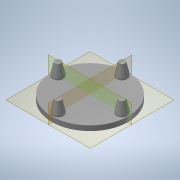
# Autodesk Inventor part: Kogel houder2
Saved by Autodesk Inventor 2021 (Build 250183000, 183)
## iProperties
Manager: PJ / DCS
Company: Emmaüs Bovenbouw Aalter
Created: 2021-02-11
Part Number: Kogel houder2
Material: S235
Catalog Web Link: http://emmausbovenbouw.op-weg.be/
Vendor: Emmaüsinstituut Bovenbouw Aalter
Document SubType Name: Modeling
Designer: Antho
Engineer: Declercq St.
Manufacturer: Standard
Standards Organization: Custom
Density: 7.86 g/cm^3
Appearance: Steel
Title: Algemene titel
Subject: Specifieke titel
Author: Antho
Keywords: Ruwe Ø xxxxx
Comments: Opmerking
Autodesk Inventor part; units mm, degrees
sketch "Sketch1" plane through (0, 0, 0) normal (0, 0, 1) x (1, 0, 0)
  line L0 (0, 2.5316) -> (0, -2.5316) construction
  line L1 (-5.1172, 0) -> (5.1172, 0) construction
  circle A0 centre (0, 0) radius 15.5
  dimension "d0" = 31
  constraints: 4 end point, 2 coincident, 2 midpoint, 1 centre point, 1 horizontal, 1 vertical
  measures "d0" diameter of A0
extrude "Extrusion1" add sketch "Sketch1" along normal blind 2
sketch "Sketch2" plane through (0, 0, 2) normal (0, 0, 1) x (1, 0, 0)
  circle A0 centre (0, 0) radius 13
  line L0 (0, 0) -> (0, 13)
  line L1 (0, 0) -> (13, 0)
  line L2 (0, 0) -> (0, -13)
  line L3 (0, 0) -> (-13, 0)
  circle A1 centre (-13, 0) radius 2.25
  circle A2 centre (0, 13) radius 2.25
  circle A3 centre (13, 0) radius 2.25
  circle A4 centre (0, -13) radius 2.25
  dimension "d3" = 26
  dimension "d4" = 4.5
  dimension "d5" = 4.5
  dimension "d6" = 4.5
  dimension "d7" = 4.5
  constraints: 8 end point, 5 centre point, 5 coincident, 4 point on circle, 2 point on line, 1 perpendicular, 1 vertical
  measures "d3" diameter of A0
  measures "d4" diameter of A1
  measures "d5" diameter of A2
  measures "d6" diameter of A3
  measures "d7" diameter of A4
extrude "Extrusion2" add sketch "Sketch2" along normal blind 5 contours L1 A3 A0 | A0 A3 | A0 A3 L1 | A2 L0 A0 | A0 A2 | A4 A0 | A0 L2 A4 | L0 A2 A0 | A0 A4 L2 | A1 A0 L3 | L3 A0 A1 | A0 A1
chamfer "Chamfer1" distance 1 distance2 4.5 1 edges at (-15.25, 0, 7) measured on face at (-13.6641, 0.3485, 7)
chamfer "Chamfer2" distance 1 distance2 4.5 1 edges at (-2.25, -13, 7) measured on face at (-0.0904, -12.342, 7)
chamfer "Chamfer3" distance 1 distance2 4.5 1 edges at (10.75, 0, 7) measured on face at (12.3359, 0.3485, 7)
chamfer "Chamfer4" distance 1 distance2 4.5 1 edges at (-2.25, 13, 7) measured on face at (-0.0904, 13.658, 7)
body "Solid1"
